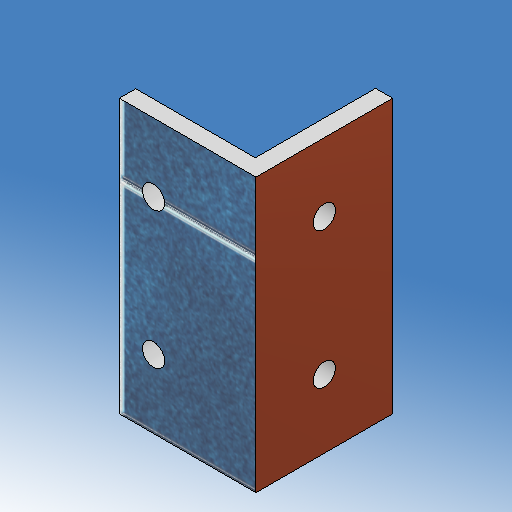
# Autodesk Inventor part: LBracketConnectors
Saved by Autodesk Inventor 2025 (Build 290162000, 162)
## iProperties
Created: 2024-06-15
Part Number: LBracketConnectors
Material: Generic
Document SubType Name: Modeling
Designer: seene
Density: 1 g/cm^3
Appearance: Default
Author: seene
Autodesk Inventor part; units mm, degrees
ref_plane "YZ Plane" through (0, 0, 0) normal (1, 0, 0) x (0, 1, 0)
ref_plane "XZ Plane" through (0, 0, 0) normal (0, 1, 0) x (-1, 0, 0)
ref_plane "XY Plane" through (0, 0, 0) normal (0, 0, 1) x (1, 0, 0)
sketch "Sketch1" plane through (0, 0, 0) normal (0, 1, 0) x (-1, 0, 0)
  line L0 (0, 0) -> (0, -25.4)
  line L1 (0, -25.4) -> (0, 0)
  line L2 (0, 0) -> (25.4, 0)
  line L3 (25.4, 0) -> (25.4, -3.048)
  line L4 (25.4, -3.048) -> (3.175, -3.048)
  line L5 (3.175, -3.048) -> (3.175, -25.4)
  line L6 (3.175, -25.4) -> (0, -25.4)
  dimension "d0" = 25.4
  dimension "d1" = 25.4
  dimension "d2" = 3.048
  dimension "d3" = 3.175
  constraints: 14 end point, 5 perpendicular, 1 collinear, 1 vertical
  measures "d0" distance of L0.start L0.end
  measures "d1" distance of L0.start L2.end
  measures "d2" distance of L2.end L3.end
  measures "d3" distance of L5.end L0.end
extrude "Extrusion1" add sketch "Sketch1" along normal blind 50.8
sketch "Sketch2" plane through (-25.4, 0, 0) normal (0, 0, 1) x (1, 0, 0)
  line L0 (22.225, 50.8) -> (0, 50.8) construction
  line L1 (22.225, 0) -> (0, 0) construction
  line L2 (6.35, 50.8) -> (6.35, 0) construction
  line L3 (0, 0) -> (0, 50.8) construction
  circle A0 centre (6.35, 12.7) radius 2.0701
  circle A1 centre (6.35, 38.1) radius 2.0701
  line L4 (25.4, 0) -> (25.4, 50.8) projected
  dimension "d7" = 4.1402
  dimension "d8" = 4.1402
  dimension "d9" = 25.4
  dimension "d10" = 12.7
  dimension "d16" = 19.05
  constraints: 4 point on line, 2 centre point, 2 end point, 1 vertical
  measures "d7" diameter of A0
  measures "d8" diameter of A1
  measures "d9" distance of A0.centre A1.centre
  measures "d10" distance from line of L1 A0.centre
  measures "d16" distance from line of L4 A0.centre
sketch "Sketch3" plane through (0, 0, 0) normal (1, 0, 0) x (0, 0, -1)
  line L0 (0, 0) -> (25.4, 0) projected
  line L1 (25.4, 0) -> (25.4, 50.8) projected
  line L2 (0, 50.8) -> (25.4, 50.8) projected
  line L3 (0, 0) -> (0, 50.8) projected
  circle A0 centre (12.7, 38.1) radius 2.0701
  circle A1 centre (12.7, 12.7) radius 2.0701
  dimension "d11" = 4.1402
  dimension "d12" = 4.1402
  dimension "d13" = 12.7
  dimension "d14" = 12.7
  dimension "d15" = 25.4
  constraints: 2 centre point, 1 vertical alignment
  measures "d11" diameter of A0
  measures "d12" diameter of A1
  measures "d13" distance from line of A0.centre L3
  measures "d14" distance from line of L2 A0.centre
  measures "d15" distance of A0.centre A1.centre
extrude "Extrusion2" cut sketch "Sketch2" against normal through all
extrude "Extrusion3" cut sketch "Sketch3" against normal blind 25.4 contours A0 | A1
body "Solid1"
